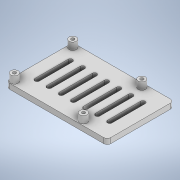
# Autodesk Inventor part: Base Rev A
Saved by Autodesk Inventor 2021 (Build 250183000, 183)
## iProperties
Created: 2020-10-18
Part Number: Base Rev A
Material: Generic
Document SubType Name: Modeling
Designer: cmzgt
Density: 1 g/cm^3
Appearance: Default
Author: cmzgt
## iProperties of the stored document _3DPrint.ipt
Created: 2020-10-18
Part Number: _3DPrint
Material: Generic
Document SubType Name: Modeling
Designer: cmzgt
Density: 1 g/cm^3
Appearance: Default
Author: cmzgt
Autodesk Inventor part; units mm, degrees
ref_plane "YZ Plane" through (0, 0, 0) normal (1, 0, 0) x (0, 1, 0)
ref_plane "XZ Plane" through (0, 0, 0) normal (0, 1, 0) x (-1, 0, 0)
ref_plane "XY Plane" through (0, 0, 0) normal (0, 0, 1) x (1, 0, 0)
sketch "Sketch1" plane through (0, 0, 0) normal (0, 1, 0) x (-1, 0, 0)
  line L0 (-42.5, -28) -> (42.5, -28)
  line L1 (42.5, -28) -> (42.5, 28)
  line L2 (42.5, 28) -> (-42.5, 28)
  line L3 (-42.5, 28) -> (-42.5, -28)
  line L4 (-42.5, -28) -> (42.5, 28) construction
  line L5 (42.5, -28) -> (-42.5, 28) construction
  point P0 (0, 0)
  dimension "d0" = 85
  dimension "d1" = 56
  constraints: 12 end point, 2 midpoint, 2 parallel, 1 horizontal, 1 perpendicular
  measures "d0" distance of L2.end L1.end
  measures "d1" distance of L1.end L0.end
extrude "Extrusion1" add sketch "Sketch1" along normal blind 4.445
sketch "Sketch2" plane through (0, 4.445, 0) normal (0, 1, 0) x (1, 0, 0)
  circle A0 centre (-39, -24.5) radius 1.375
  circle A1 centre (-39, -24.5) radius 3.1
  line L0 (-42.5, -28) -> (42.5, -28) projected
  line L1 (-42.5, 28) -> (-42.5, -28) projected
  line L2 (-42.5, 0) -> (42.5, 0)
  line L3 (42.5, -28) -> (42.5, 28) projected
  line L4 (0, 28) -> (0, -28)
  circle A2 centre (-39, 24.5) radius 1.375
  circle A3 centre (-39, 24.5) radius 3.1
  circle A4 centre (19, 24.5) radius 1.375
  circle A5 centre (19, 24.5) radius 3.1
  circle A6 centre (19, -24.5) radius 3.1
  circle A7 centre (19, -24.5) radius 1.375
  line L5 (42.5, 28) -> (-42.5, 28) projected
  point P0 (0, 0)
  dimension "d4" = 2.75
  dimension "d5" = 6.2
  dimension "d6" = 3.5
  dimension "d7" = 3.5
  dimension "d30" = 6.2
  dimension "d31" = 2.75
  dimension "d32" = 58
  dimension "d33" = 3.5
  constraints: 8 centre point, 4 coincident, 4 end point, 4 symmetric about line, 3 midpoint, 4 other
  measures "d4" diameter of A0
  measures "d5" diameter of A1
  measures "d6" distance from line of L0 A0.centre
  measures "d7" distance from line of L1 A0.centre
  measures "d30" diameter of A5
  measures "d31" diameter of A4
  measures "d32" distance of A2.centre A5.centre
  measures "d33" distance from line of L5 A5.centre
fillet "Fillet2" radius 3 4 edges at (42.5, 2.2225, 28) (-42.5, 2.2225, 28) (42.5, 2.2225, -28) (-42.5, 2.2225, -28)
extrude "Extrusion2" add sketch "Sketch2" along normal blind 6.0706 contours A1 | A3 | A5 | A6
sketch "Sketch4" plane through (0, 4.445, 0) normal (0, 1, 0) x (1, 0, 0)
  line L0 (0, -13.97) -> (0, 13.97) construction
  line L1 (1.905, -13.97) -> (1.905, 13.97)
  line L2 (-1.905, 13.97) -> (-1.905, -13.97)
  arc A0 (-1.905, -13.97) -> (1.905, -13.97) centre (0, -13.97) ccw
  arc A1 (1.905, 13.97) -> (-1.905, 13.97) centre (0, 13.97) ccw
  line L3 (39.5, 28) -> (-39.5, 28) construction
  line L4 (0, 28) -> (0, -28) construction
  line L5 (-39.5, -28) -> (39.5, -28) construction
  line L6 (42.5, -25) -> (42.5, 25) construction
  line L7 (42.5, 0) -> (-42.5, 0) construction
  line L8 (-42.5, 25) -> (-42.5, -25) construction
  line L9 (-8.255, -13.97) -> (-8.255, 13.97)
  line L10 (-12.065, 13.97) -> (-12.065, -13.97)
  arc A2 (-8.255, 13.97) -> (-12.065, 13.97) centre (-10.16, 13.97) ccw
  arc A3 (-12.065, -13.97) -> (-8.255, -13.97) centre (-10.16, -13.97) ccw
  line L11 (-18.415, -13.97) -> (-18.415, 13.97)
  line L12 (-22.225, 13.97) -> (-22.225, -13.97)
  arc A4 (-18.415, 13.97) -> (-22.225, 13.97) centre (-20.32, 13.97) ccw
  arc A5 (-22.225, -13.97) -> (-18.415, -13.97) centre (-20.32, -13.97) ccw
  line L13 (-28.575, -13.97) -> (-28.575, 13.97)
  line L14 (-32.385, 13.97) -> (-32.385, -13.97)
  arc A6 (-28.575, 13.97) -> (-32.385, 13.97) centre (-30.48, 13.97) ccw
  arc A7 (-32.385, -13.97) -> (-28.575, -13.97) centre (-30.48, -13.97) ccw
  line L15 (12.065, -13.97) -> (12.065, 13.97)
  line L16 (8.255, 13.97) -> (8.255, -13.97)
  arc A8 (12.065, 13.97) -> (8.255, 13.97) centre (10.16, 13.97) ccw
  arc A9 (8.255, -13.97) -> (12.065, -13.97) centre (10.16, -13.97) ccw
  line L17 (1.905, -13.97) -> (1.905, 13.97)
  line L18 (-1.905, 13.97) -> (-1.905, -13.97)
  arc A10 (1.905, 13.97) -> (-1.905, 13.97) centre (0, 13.97) ccw
  arc A11 (-1.905, -13.97) -> (1.905, -13.97) centre (0, -13.97) ccw
  line L19 (-8.255, -13.97) -> (-8.255, 13.97)
  line L20 (-12.065, 13.97) -> (-12.065, -13.97)
  arc A12 (-8.255, 13.97) -> (-12.065, 13.97) centre (-10.16, 13.97) ccw
  arc A13 (-12.065, -13.97) -> (-8.255, -13.97) centre (-10.16, -13.97) ccw
  line L21 (-18.415, -13.97) -> (-18.415, 13.97)
  line L22 (-22.225, 13.97) -> (-22.225, -13.97)
  arc A14 (-18.415, 13.97) -> (-22.225, 13.97) centre (-20.32, 13.97) ccw
  arc A15 (-22.225, -13.97) -> (-18.415, -13.97) centre (-20.32, -13.97) ccw
  line L23 (22.225, -13.97) -> (22.225, 13.97)
  line L24 (18.415, 13.97) -> (18.415, -13.97)
  arc A16 (22.225, 13.97) -> (18.415, 13.97) centre (20.32, 13.97) ccw
  arc A17 (18.415, -13.97) -> (22.225, -13.97) centre (20.32, -13.97) ccw
  line L25 (12.065, -13.97) -> (12.065, 13.97)
  line L26 (8.255, 13.97) -> (8.255, -13.97)
  arc A18 (12.065, 13.97) -> (8.255, 13.97) centre (10.16, 13.97) ccw
  arc A19 (8.255, -13.97) -> (12.065, -13.97) centre (10.16, -13.97) ccw
  line L27 (1.905, -13.97) -> (1.905, 13.97)
  line L28 (-1.905, 13.97) -> (-1.905, -13.97)
  arc A20 (1.905, 13.97) -> (-1.905, 13.97) centre (0, 13.97) ccw
  arc A21 (-1.905, -13.97) -> (1.905, -13.97) centre (0, -13.97) ccw
  line L29 (-8.255, -13.97) -> (-8.255, 13.97)
  line L30 (-12.065, 13.97) -> (-12.065, -13.97)
  arc A22 (-8.255, 13.97) -> (-12.065, 13.97) centre (-10.16, 13.97) ccw
  arc A23 (-12.065, -13.97) -> (-8.255, -13.97) centre (-10.16, -13.97) ccw
  line L31 (32.385, -13.97) -> (32.385, 13.97)
  line L32 (28.575, 13.97) -> (28.575, -13.97)
  arc A24 (32.385, 13.97) -> (28.575, 13.97) centre (30.48, 13.97) ccw
  arc A25 (28.575, -13.97) -> (32.385, -13.97) centre (30.48, -13.97) ccw
  line L33 (22.225, -13.97) -> (22.225, 13.97)
  line L34 (18.415, 13.97) -> (18.415, -13.97)
  arc A26 (22.225, 13.97) -> (18.415, 13.97) centre (20.32, 13.97) ccw
  arc A27 (18.415, -13.97) -> (22.225, -13.97) centre (20.32, -13.97) ccw
  line L35 (12.065, -13.97) -> (12.065, 13.97)
  line L36 (8.255, 13.97) -> (8.255, -13.97)
  arc A28 (12.065, 13.97) -> (8.255, 13.97) centre (10.16, 13.97) ccw
  arc A29 (8.255, -13.97) -> (12.065, -13.97) centre (10.16, -13.97) ccw
  line L37 (1.905, -13.97) -> (1.905, 13.97)
  line L38 (-1.905, 13.97) -> (-1.905, -13.97)
  arc A30 (1.905, 13.97) -> (-1.905, 13.97) centre (0, 13.97) ccw
  arc A31 (-1.905, -13.97) -> (1.905, -13.97) centre (0, -13.97) ccw
  point P0 (0, 0)
  dimension "d18" = 13.97
  dimension "d19" = 3.81
  dimension "d22" = 10.16
  dimension "d25" = 10.16
  constraints: 72 end point, 64 point on circle, 32 centre point, 5 midpoint, 4 tangent, 2 horizontal, 1 parallel, 1 vertical, 150 other
  measures "d18" distance of point (0, 0) L0.end
  measures "d19" diameter of A1
  measures "d22" distance of L1.start L9.start
  measures "d25" distance of L1.start L15.start
extrude "Extrusion3" cut sketch "Sketch4" against normal blind 4.445
body "Solid1"
